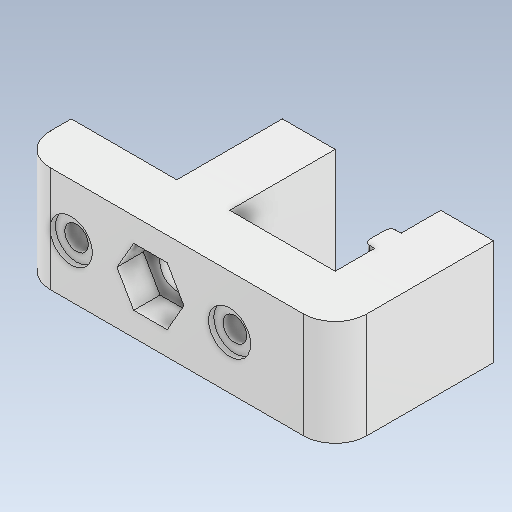
# Autodesk Inventor part: ZItemMountCable
Saved by Autodesk Inventor 2020 (Build 240168000, 168)
## iProperties
Created: 2022-03-24
Part Number: ZItemMountCable
Material: Tworzywo sztuczne ABS
Document SubType Name: Modeling
Designer: mikoma
Density: 1.06 g/cm^3
Appearance: Gładki — biały
Mass: 19.2306 g
Surface Area: 72.2385 cm^2
Volume: 18.1421 cm^3
Author: mikoma
Autodesk Inventor part; units mm, degrees
ref_plane "YZ Plane" through (0, 0, 0) normal (1, 0, 0) x (0, 1, 0)
ref_plane "XZ Plane" through (0, 0, 0) normal (0, 1, 0) x (-1, 0, 0)
ref_plane "XY Plane" through (0, 0, 0) normal (0, 0, 1) x (1, 0, 0)
sketch "Szkic1" plane through (0, 0, 0) normal (0, 1, 0) x (-1, 0, 0)
  line L0 (25, 20) -> (5, 20)
  line L1 (5, 20) -> (5, 0)
  line L2 (5, 0) -> (25, 0)
  line L3 (25, 0) -> (25, 20)
  line L4 (-5, 20) -> (-25, 20)
  line L5 (-25, 20) -> (-25, 0)
  line L6 (-25, 0) -> (-5, 0)
  line L7 (-5, 0) -> (-5, 20)
  line L8 (25, 0) -> (-25, 0)
  line L9 (-25, 0) -> (-25, 30)
  line L10 (-25, 30) -> (25, 30)
  line L11 (25, 30) -> (25, 0)
  line L12 (-25, 30) -> (-35, 30)
  line L13 (-35, 30) -> (-35, 0)
  line L14 (-35, 0) -> (-25, 0)
  line L15 (-25, 0) -> (-25, 30)
  line L16 (-25, 12.5) -> (-24, 12.5)
  line L17 (-23, 11.5) -> (-23, 8.5)
  line L18 (-24, 7.5) -> (-25, 7.5)
  line L19 (-25, 7.5) -> (-25, 12.5)
  arc A0 (-23, 11.5) -> (-24, 12.5) centre (-24, 11.5) ccw
  arc A1 (-24, 7.5) -> (-23, 8.5) centre (-24, 8.5) ccw
  point P0 (0, 0)
  point P1 (-15, 20)
  point P2 (15, 20)
  point P3 (15, 0)
  point P4 (-5, 0)
  point P5 (5, 0)
  point P6 (-23, 7.5)
  point P7 (-23, 12.5)
  dimension "d0" = 20
  dimension "d1" = 20
  dimension "d2" = 20
  dimension "d3" = 20
  dimension "d4" = 50
  dimension "d5" = 25
  dimension "d6" = 10
  dimension "d28" = 10
  dimension "d29" = 5
  dimension "d30" = 7.5
  dimension "d31" = 2
  dimension "d33" = 1
  constraints: 40 end point, 10 parallel, 5 horizontal, 5 perpendicular, 5 point on line, 4 point on circle, 4 tangent, 3 horizontal alignment, 3 midpoint, 2 centre point, 1 equal radius, 1 vertical alignment
  measures "d0" distance of L2.end L0.start
  measures "d1" distance of L1.end L2.end
  measures "d2" distance of L6.end L4.start
  measures "d3" distance of L5.end L6.end
  measures "d4" distance between parallel lines of L5 L3
  measures "d5" distance from line of point (0, 0) L3
  measures "d6" distance between parallel lines of L0 L10
  measures "d28" distance of L13.end L14.end
  measures "d29" distance between parallel lines of L18 L16
  measures "d30" distance between parallel lines of L8 L18
  measures "d31" distance between parallel lines of L5 L17
  measures "d33" radius of A0
extrude "Wyciągnięcie proste1" add sketch "Szkic1" along normal blind 20 contours L0 L1 L8 L7 L4 L9 L10 L11 | L9 L5 L14 L13 L12 | L16 A0 L17 A1 L18 L5
sketch "Szkic2" plane through (5, 0, 0) normal (0, 0, -1) x (-1, 0, 0)
  circle A0 centre (5, 10) radius 3.25
  circle A1 centre (20, 10) radius 2.25
  circle A2 centre (-10, 10) radius 2.25
  line L0 (0, 0) -> (0, 20) projected
  line L1 (0, 0) -> (10, 0) projected
  line L2 (-20, 0) -> (0, 0) projected
  line L3 (30, 0) -> (30, 20) projected
  circle A3 centre (-10, 10) radius 4
  circle A4 centre (20, 10) radius 4
  line L4 (1.8246, 15.5) -> (8.1754, 15.5)
  line L5 (8.1754, 15.5) -> (11.3509, 10)
  line L6 (11.3509, 10) -> (8.1754, 4.5)
  line L7 (8.1754, 4.5) -> (1.8246, 4.5)
  line L8 (1.8246, 4.5) -> (-1.3509, 10)
  line L9 (-1.3509, 10) -> (1.8246, 15.5)
  line L10 (-20, 0) -> (-20, 20) projected
  point P0 (5, 0)
  dimension "d9" = 6.5
  dimension "d10" = 5
  dimension "d11" = 10
  dimension "d13" = 10
  dimension "d14" = 10
  dimension "d15" = 4.5
  dimension "d16" = 4.5
  dimension "d20" = 8
  dimension "d21" = 8
  dimension "d25" = 11
  dimension "d32" = 10
  constraints: 12 end point, 5 centre point, 3 coincident, 1 horizontal, 1 horizontal alignment, 13 other
  measures "d9" diameter of A0
  measures "d10" distance from line of A0.centre L0
  measures "d11" distance from line of L1 A0.centre
  measures "d13" distance from line of A2.centre L2
  measures "d14" distance from line of L3 A1.centre
  measures "d15" diameter of A2
  measures "d16" diameter of A1
  measures "d20" diameter of A3
  measures "d21" diameter of A4
  measures "d25" distance between parallel lines of L7 L4
  measures "d32" distance from line of L10 A2.centre
extrude "Wyciągnięcie proste2" cut sketch "Szkic2" against normal through all contours A0 | A1 | A2
extrude "Wyciągnięcie proste3" cut sketch "Szkic2" along normal blind 5 from surface at -30 contours A0 | L8 L9 L0 | L0 L9 L4 L5 L6 L7 L8
fillet "Zaokrąglenie1" radius 6 2 edges at (-25, 10, 30) (35, 10, 30)
extrude "Wyciągnięcie proste4" cut sketch "Szkic2" along normal blind 1 from surface at -30 contours A1 | A2 | A3 | A4
